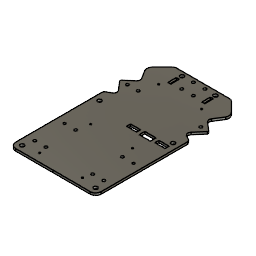
base_piso_1_mot_ack (Autodesk Fusion 360 design; units mm, degrees)
Autodesk Fusion 360 part; units mm, degrees
imported_body "Operación base derivada4" makes body 1
imported_body "Operación base derivada5" makes body 2
imported_body "Operación base derivada6" makes body 3
imported_body "Operación base derivada7" makes body 4
imported_body "Operación base derivada8" makes body 5
sketch "Boceto1" plane through (0, 0, 0) normal (0, 0, 1) x (1, 0, 0)
  circle A0 centre (-65.6693, 15.1765) radius 3.5
  circle A1 centre (-65.5152, 65.1825) radius 2.5
  circle A2 centre (-38.1168, -120.0235) radius 1.5
  circle A3 centre (-46.2152, 65.1825) radius 2.5
  circle A4 centre (-61.586, -51.7549) radius 2.1
  line L0 (-66.185, 38.9484) -> (-74.3516, 34.3123)
  circle A5 centre (-65.6693, -123.8667) radius 3.4995
  circle A6 centre (-41.586, -51.7549) radius 2.5
  circle A7 centre (-37.1767, -29.3011) radius 1.5
  arc A8 (-47.3019, 135.1765) -> (-52.9552, 132.8333) centre (-47.2992, 127.1786) ccw
  line L1 (-72.3166, 102.958) -> (-62.2876, 87.2513)
  arc A9 (-74.3516, 34.3123) -> (-76.6693, 30.4647) centre (-72.1596, 30.3701) ccw
  line L2 (-78.4139, 63.8607) -> (-65.0156, 48.214)
  line L3 (-63.4701, 79.2819) -> (-78.1886, 66.7247)
  line L4 (-52.9552, 132.8333) -> (-70.2152, 115.5734)
  circle A10 centre (-29.6701, 127.1824) radius 3.5
  arc A11 (-78.1886, 66.7247) -> (-78.4139, 63.8607) centre (-76.8581, 65.1792) ccw
  circle A12 centre (-61.586, -105.2549) radius 2.5
  arc A13 (-76.6693, -124.8933) -> (-66.6474, -134.8235) centre (-66.6656, -124.8196) ccw
  circle A14 centre (-41.586, -105.2549) radius 2.5
  line L5 (-76.6693, 30.4647) -> (-76.6693, -124.8933)
  arc A15 (-65.0156, 48.214) -> (-66.185, 38.9484) centre (-69.1038, 44.0234) cw
  arc A16 (-70.2152, 115.5734) -> (-72.3166, 102.958) centre (-62.4371, 107.7951) ccw
  arc A17 (-62.2876, 87.2513) -> (-63.4701, 79.2819) centre (-67.4637, 83.9469) cw
  line L6 (0.3307, 135.1924) -> (0.3307, -134.702) construction
  line L7 (-95, 0) -> (105, 0) construction
  line L8 (-47.3019, 135.1765) -> (0.3307, 135.1924)
  line L9 (-66.6474, -134.8235) -> (0.3307, -134.702)
  circle A18 centre (30.3316, 127.1824) radius 3.5
  arc A19 (53.6167, 132.8333) -> (47.9634, 135.1765) centre (47.9607, 127.1786) ccw
  line L10 (0.3307, 135.1924) -> (0.3307, -134.702) construction
  line L11 (53.6167, 132.8333) -> (70.8766, 115.5734)
  arc A20 (72.978, 102.958) -> (70.8766, 115.5734) centre (63.0985, 107.7951) ccw
  arc A21 (79.0754, 63.8607) -> (78.8501, 66.7247) centre (77.5195, 65.1792) ccw
  arc A22 (77.3307, 30.4647) -> (75.013, 34.3123) centre (72.8211, 30.3701) ccw
  line L12 (64.1316, 79.2819) -> (78.8501, 66.7247)
  circle A23 centre (66.1766, 65.1825) radius 2.5
  line L13 (47.9634, 135.1765) -> (0.3307, 135.1924)
  line L14 (79.0754, 63.8607) -> (65.677, 48.214)
  circle A24 centre (66.3307, -123.8667) radius 3.4995
  circle A25 centre (38.7783, -120.0235) radius 1.5
  circle A26 centre (42.2474, -105.2549) radius 2.5
  circle A27 centre (66.3307, 15.1765) radius 3.5
  arc A28 (67.3089, -134.8235) -> (77.3307, -124.8933) centre (67.327, -124.8196) ccw
  line L15 (72.978, 102.958) -> (62.949, 87.2513)
  line L16 (66.8464, 38.9484) -> (75.013, 34.3123)
  arc A29 (66.8464, 38.9484) -> (65.677, 48.214) centre (69.7652, 44.0234) cw
  circle A30 centre (62.2474, -51.7549) radius 2.1
  circle A31 centre (37.8381, -29.3011) radius 1.5
  line L17 (67.3089, -134.8235) -> (0.3307, -134.702)
  line L18 (77.3307, 30.4647) -> (77.3307, -124.8933)
  arc A32 (64.1316, 79.2819) -> (62.949, 87.2513) centre (68.1251, 83.9469) cw
  circle A33 centre (62.2474, -105.2549) radius 2.5
  circle A34 centre (42.2474, -51.7549) radius 2.5
  circle A35 centre (-10.0983, 128.1179) radius 2.5
  circle A36 centre (-10.0983, 107.2599) radius 2.5
  circle A37 centre (10.7597, 128.1179) radius 2.5
  circle A38 centre (10.7597, 107.2599) radius 2.5
  line L19 (22.8307, -2.1499) -> (42.8307, -2.1499)
  line L20 (49.3307, -0.3235) -> (67.3307, 6.6765) construction
  line L21 (22.8307, 7.8501) -> (22.8307, -2.1499)
  line L22 (42.8307, -2.1499) -> (42.8307, 7.8501)
  line L23 (42.8307, 7.8501) -> (22.8307, 7.8501)
  line L24 (67.3307, -0.3235) -> (49.3307, -0.3235)
  line L25 (-1.6693, -0.3235) -> (16.3307, 6.6765) construction
  line L26 (16.3307, -0.3235) -> (-1.6693, 6.6765) construction
  line L27 (16.3307, -0.3235) -> (-1.6693, -0.3235)
  line L28 (49.3307, -0.3235) -> (49.3307, 6.6765)
  line L29 (67.3307, 6.6765) -> (67.3307, -0.3235)
  line L30 (67.3307, -0.3235) -> (49.3307, 6.6765) construction
  line L31 (-1.6693, -0.3235) -> (-1.6693, 6.6765)
  line L32 (16.3307, 6.6765) -> (16.3307, -0.3235)
  line L33 (-1.6693, 6.6765) -> (16.3307, 6.6765)
  line L34 (49.3307, 6.6765) -> (67.3307, 6.6765)
  circle A39 centre (39.0308, 93.7385) radius 1.5
  circle A40 centre (46.8577, 65.1973) radius 2.5
  circle A41 centre (46.8577, 65.1973) radius 2.5
  circle A42 centre (-38.3694, 93.7385) radius 1.5
  line L35 (-32.6693, 120) -> (-27.6693, 120)
  line L36 (-27.6693, 120) -> (-27.6693, 105)
  line L37 (-27.6693, 105) -> (-32.6693, 105)
  line L38 (-32.6693, 105) -> (-32.6693, 120)
  line L39 (28.3307, 120) -> (28.3307, 105)
  line L40 (28.3307, 105) -> (33.3307, 105)
  line L41 (33.3307, 105) -> (33.3307, 120)
  line L42 (33.3307, 120) -> (28.3307, 120)
  line L43 (27.6693, -120) -> (27.6693, -105)
  point P0 (-30.5142, -346.9358)
  point P1 (7.3307, 3.1765)
  point P2 (58.3307, 3.1765)
  dimension "d241" = 270
  dimension "d242" = 7
  dimension "d243" = 5
  dimension "d244" = 5
  dimension "d245" = 7
  dimension "d247" = 46.5459
  dimension "d248" = 19.3
  dimension "d249" = 11.3429
  dimension "d250" = 41.9167
  dimension "d251" = 20
  dimension "d252" = 41.9167
  dimension "d253" = 20
  dimension "d254" = 38.4476
  dimension "d255" = 37.5074
  dimension "d256" = 29.3011
  dimension "d257" = 51.7549
  dimension "d258" = 105.2549
  dimension "d259" = 120.0235
  dimension "d260" = 11
  dimension "d261" = 11.0004
  dimension "d264" = 10.429
  dimension "d266" = 7.071
  dimension "d267" = 20.858
  dimension "d268" = 10.429
  dimension "d269" = 8
  dimension "d270" = 77
  dimension "d275" = 18
  dimension "d276" = 7
  dimension "d277" = 20
  dimension "d278" = 10
  dimension "d279" = 18
  dimension "d280" = 7
  dimension "d285" = 132
  dimension "d287" = 11
  dimension "d288" = 10
  dimension "d291" = 6.5
  dimension "d292" = 6.5
  dimension "d293" = 28
  constraint horizontal L7
  constraint tangent A8 L8
  constraint tangent A13 L9
  constraint symmetric L0.end L6 A22.end
  constraint symmetric A9.end L6 A22.start
  constraint symmetric A13.end L6 A28.start
  constraint symmetric A8.end L6 A19.start
  constraint symmetric A8.start L6 A19.end
  constraint symmetric L3.end L6 A21.end
  constraint symmetric L3.start L6 L12.start
  constraint symmetric A13.start L6 A28.end
  constraint symmetric L0.start L6 L16.start
  constraint symmetric L2.start L6 A21.start
  constraint symmetric L2.end L6 L14.end
  constraint symmetric L4.end L6 L11.end
  constraint symmetric L1.end L6 L15.end
  constraint symmetric L1.start L6 A20.start
  constraint symmetric A0 L6 A27
  constraint symmetric A1 L6 A23
  constraint symmetric A2 L6 A25
  constraint symmetric A4 L6 A30
  constraint symmetric A5 L6 A24
  constraint symmetric A6 L6 A34
  constraint symmetric A7 L6 A31
  constraint symmetric A8 L6 A19
  constraint symmetric A9 L6 A22
  constraint symmetric A10 L6 A18
  constraint symmetric A11 L6 A21
  constraint symmetric A12 L6 A33
  constraint symmetric A13 L6 A28
  constraint symmetric A14 L6 A26
  constraint symmetric A15 L6 A29
  constraint symmetric A16 L6 A20
  constraint symmetric A17 L6 A32
  constraint symmetric L8.end L6 L10.start
  constraint symmetric L9.end L6 L10.end
  constraint symmetric L10 A35 A37
  constraint symmetric L10 A36 A38
  constraint horizontal L24
  constraint perpendicular L24 L28
  constraint parallel L24 L34
  constraint parallel L28 L29
  constraint coincident P2 L30
  constraint coincident P2 L20
  constraint perpendicular L22 L23
  constraint parallel L21 L22
  constraint parallel L19 L23
  constraint horizontal L27
  constraint perpendicular L27 L31
  constraint parallel L27 L33
  constraint parallel L31 L32
  constraint coincident P1 L26
  constraint coincident P1 L25
  constraint symmetric L10 A39 A42
  constraint horizontal L35
  constraint vertical L36
  constraint horizontal L37
  constraint vertical L38
  constraint symmetric L10 L35.start L41.end
  constraint symmetric L10 L35.end L39.start
  constraint symmetric L10 L36.end L39.end
  constraint symmetric L10 L37.end L40.end
  measures "d241" vertical distance of A13.end A8.start
  measures "d242" diameter of A0
  measures "d243" diameter of A3
  measures "d244" diameter of A1
  measures "d245" diameter of A10
  measures "d247" distance of A3.centre L6
  measures "d248" distance of A1.centre A3.centre
  measures "d249" distance of A1.centre A11.centre
  measures "d250" distance of A6.centre L6
  measures "d251" distance of A4.centre A6.centre
  measures "d252" distance of A14.centre L6
  measures "d253" distance of A12.centre A14.centre
  measures "d254" distance of A2.centre L6
  measures "d255" distance of A7.centre L6
  measures "d256" distance of A7.centre L7
  measures "d257" distance of A6.centre L7
  measures "d258" distance of A14.centre L7
  measures "d259" distance of A2.centre L7
  measures "d260" distance of A5.centre L5
  measures "d261" distance of A13.end A5.centre
  measures "d264" distance of L10 A35.centre
  measures "d266" distance of L8 A35.centre
  measures "d267" vertical distance of A36.centre A35.centre
  measures "d268" distance of L6 A36.centre
  measures "d269" distance of A10.centre L8
  measures "d270" distance of L5 L10
  measures "d275" distance of L28.end L20.end
  measures "d276" distance of L28.end L20.start
  measures "d277" distance of L22.end L21.start
  measures "d278" distance of L21.start L19.start
  measures "d279" distance of L25.end L26.end
  measures "d280" distance of L25.start L26.end
  measures "d285" vertical distance of A19.end P2
  measures "d287" distance of A0.centre L5
  measures "d288" distance of L18 L29
  measures "d291" distance of L22 L28
  measures "d292" distance of L21 L32
  measures "d293" distance of L6 L36
extrude "Extruir7" add sketch "Boceto1" along normal blind 4 separate body contours L0 A8 L1 A9 L2 L3 L4 A11 A13 L5 A15 A16 A17 L8 L9 A19 L11 A20 A21 A22 L12 L13 L14 A28 L15 L16 A29 L17 L18 A32 | A40 A41 makes body 6
sketch "Boceto15" plane through (0, 0, 4) normal (0, 0, 1) x (-1, 0, 0)
  circle A0 centre (-10.7597, -107.2599) radius 2.5
  circle A1 centre (46.2152, -65.1825) radius 2.5
  circle A2 centre (41.586, 105.2549) radius 2.5
  circle A3 centre (-62.2474, 105.2549) radius 2.5
  circle A4 centre (65.6693, -15.1765) radius 3.5
  line L0 (-22.8307, -7.8501) -> (-42.8307, -7.8501)
  line L1 (-42.8307, -7.8501) -> (-42.8307, 2.1499)
  line L2 (-42.8307, 2.1499) -> (-22.8307, 2.1499)
  line L3 (-22.8307, 2.1499) -> (-22.8307, -7.8501)
  circle A5 centre (61.586, 105.2549) radius 2.5
  circle A6 centre (-42.2474, 105.2549) radius 2.5
  circle A7 centre (-38.7783, 120.0235) radius 1.5
  circle A8 centre (10.0983, -107.2599) radius 2.5
  circle A9 centre (65.6693, 123.8667) radius 3.4995
  circle A10 centre (-62.2474, 51.7549) radius 2.1
  circle A11 centre (-66.3307, 123.8667) radius 3.4995
  circle A12 centre (61.586, 51.7549) radius 2.1
  line L4 (1.6693, 0.3235) -> (1.6693, -6.6765)
  line L5 (1.6693, -6.6765) -> (-16.3307, -6.6765)
  line L6 (-16.3307, -6.6765) -> (-16.3307, 0.3235)
  line L7 (-16.3307, 0.3235) -> (1.6693, 0.3235)
  circle A13 centre (41.586, 51.7549) radius 2.5
  circle A14 centre (-10.7597, -128.1179) radius 2.5
  line L8 (-49.3307, 0.3235) -> (-49.3307, -6.6765)
  line L9 (-49.3307, -6.6765) -> (-67.3307, -6.6765)
  line L10 (-67.3307, -6.6765) -> (-67.3307, 0.3235)
  line L11 (-67.3307, 0.3235) -> (-49.3307, 0.3235)
  circle A15 centre (37.1767, 29.3011) radius 1.5
  circle A16 centre (-37.8381, 29.3011) radius 1.5
  circle A17 centre (-66.1766, -65.1825) radius 2.5
  circle A18 centre (38.1168, 120.0235) radius 1.5
  circle A19 centre (65.5152, -65.1825) radius 2.5
  circle A20 centre (10.0983, -128.1179) radius 2.5
  circle A21 centre (-30.3316, -127.1824) radius 3.5
  circle A22 centre (29.6701, -127.1824) radius 3.5
  circle A23 centre (-42.2474, 51.7549) radius 2.5
  circle A24 centre (-66.3307, -15.1765) radius 3.5
  arc A25 (-79.0754, -63.8607) -> (-78.8501, -66.7247) centre (-77.5195, -65.1792) ccw
  line L12 (-78.8501, -66.7247) -> (-64.1316, -79.2819)
  arc A26 (-62.949, -87.2513) -> (-64.1316, -79.2819) centre (-68.1251, -83.9469) ccw
  line L13 (-62.949, -87.2513) -> (-72.978, -102.958)
  arc A27 (-72.978, -102.958) -> (-70.8766, -115.5734) centre (-63.0985, -107.7951) ccw
  line L14 (-70.8766, -115.5734) -> (-53.6167, -132.8333)
  arc A28 (-53.6167, -132.8333) -> (-47.9634, -135.1765) centre (-47.9607, -127.1786) ccw
  line L15 (-47.9634, -135.1765) -> (-0.3307, -135.1924)
  line L16 (-0.3307, -135.1924) -> (47.3019, -135.1765)
  arc A29 (47.3019, -135.1765) -> (52.9552, -132.8333) centre (47.2992, -127.1786) ccw
  line L17 (52.9552, -132.8333) -> (70.2152, -115.5734)
  arc A30 (70.2152, -115.5734) -> (72.3166, -102.958) centre (62.4371, -107.7951) ccw
  line L18 (72.3166, -102.958) -> (62.2876, -87.2513)
  arc A31 (63.4701, -79.2819) -> (62.2876, -87.2513) centre (67.4637, -83.9469) ccw
  line L19 (63.4701, -79.2819) -> (78.1886, -66.7247)
  arc A32 (78.1886, -66.7247) -> (78.4139, -63.8607) centre (76.8581, -65.1792) ccw
  line L20 (78.4139, -63.8607) -> (65.0156, -48.214)
  arc A33 (66.185, -38.9484) -> (65.0156, -48.214) centre (69.1038, -44.0234) ccw
  line L21 (66.185, -38.9484) -> (74.3516, -34.3123)
  arc A34 (74.3516, -34.3123) -> (76.6693, -30.4647) centre (72.1596, -30.3701) ccw
  line L22 (76.6693, -30.4647) -> (76.6693, 124.8933)
  arc A35 (76.6693, 124.8933) -> (66.6474, 134.8235) centre (66.6656, 124.8196) ccw
  line L23 (66.6474, 134.8235) -> (-0.3307, 134.702)
  line L24 (-0.3307, 134.702) -> (-67.3089, 134.8235)
  arc A36 (-67.3089, 134.8235) -> (-77.3307, 124.8933) centre (-67.327, 124.8196) ccw
  line L25 (-77.3307, 124.8933) -> (-77.3307, -30.4647)
  arc A37 (-77.3307, -30.4647) -> (-75.013, -34.3123) centre (-72.8211, -30.3701) ccw
  line L26 (-75.013, -34.3123) -> (-66.8464, -38.9484)
  arc A38 (-65.677, -48.214) -> (-66.8464, -38.9484) centre (-69.7652, -44.0234) ccw
  line L27 (-65.677, -48.214) -> (-79.0754, -63.8607)
  circle A39 centre (-39.0308, -93.7385) radius 1.5
  circle A40 centre (38.3694, -93.7385) radius 1.5
  line L28 (-28.3307, -120) -> (-33.3307, -120)
  line L29 (-33.3307, -120) -> (-33.3307, -105)
  line L30 (-33.3307, -105) -> (-28.3307, -105)
  line L31 (-28.3307, -105) -> (-28.3307, -120)
  line L32 (27.6693, -105) -> (32.6693, -105)
  line L33 (32.6693, -105) -> (32.6693, -120)
  line L34 (32.6693, -120) -> (27.6693, -120)
  line L35 (27.6693, -120) -> (27.6693, -105)
hidden bodies 1 2 3 4 5
named bodies: "Cuerpo1 (Contexto3)", "Cuerpo1 (1) (Contexto3)", "Cuerpo1 (2) (Contexto3)", "Cuerpo1 (3) (Contexto3)", "Cuerpo1 (4) (Contexto3)"
